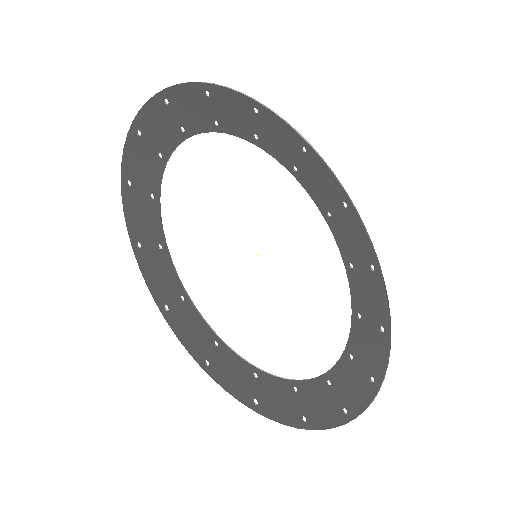
# Autodesk Inventor part: cover plate
Saved by Autodesk Inventor 2022 (Build 260148000, 148)
## iProperties
Created: 2007-05-11
Part Number: cover plate
Material: Steel, Mild
Document SubType Name: Modeling
Designer: LionelF
Density: 7.86 g/cm^3
Mass: 7586.89 g
Surface Area: 6281.43 cm^2
Volume: 965.253 cm^3
Appearance: Steel
Author: LionelF
Autodesk Inventor part; units mm, degrees
ref_plane "YZ Plane" through (0, 0, 0) normal (1, 0, 0) x (0, 1, 0)
ref_plane "XZ Plane" through (0, 0, 0) normal (0, 1, 0) x (-1, 0, 0)
ref_plane "XY Plane" through (0, 0, 0) normal (0, 0, 1) x (1, 0, 0)
sketch "Sketch1" plane through (0, 0, 0) normal (0, 0, 1) x (1, 0, 0)
  circle A0 centre (0, 0) radius 447.675
  circle A1 centre (0, 0) radius 319.0875
  dimension "d0" = 895.35
  dimension "d1" = 638.175
  constraints: 2 centre point, 1 concentric
  measures "d0" diameter of A0
  measures "d1" diameter of A1
extrude "Extrusion1" add sketch "Sketch1" along normal blind 3.175
sketch "Sketch2" plane through (0, 0, 3.175) normal (0, 0, 1) x (1, 0, 0)
  circle A0 centre (0, 0) radius 319.0875 projected
  circle A1 centre (0, 0) radius 447.675 projected
  circle A2 centre (342.9, 0) radius 7.1437
  circle A3 centre (419.1, 0) radius 7.9375
  dimension "d4" = 14.2875
  dimension "d5" = 15.875
  dimension "d6" = 342.9
  dimension "d7" = 0
  dimension "d10" = 0
  dimension "d11" = 419.1
  constraints: 2 centre point
  measures "d4" diameter of A2
  measures "d5" diameter of A3
  measures "d6" distance of A0.centre A2.centre
  measures "d7" vertical distance of A0.centre A2.centre
  measures "d10" vertical distance of A1.centre A3.centre
  measures "d11" distance of A0.centre A3.centre
extrude "Extrusion2" cut sketch "Sketch2" against normal blind 3.175 contours A2 | A3
pattern_circular "Circular Pattern1" count 16 over 360 about axis through (0, 0, 0) along (0, 0, 1) of "Extrusion2"
body "Solid1"
